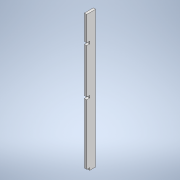
# Autodesk Inventor part: sideHolder
Saved by Autodesk Inventor 2020 (Build 240168000, 168)
## iProperties
Created: 2022-03-24
Part Number: sideHolder
Material: Pappel
Document SubType Name: Modeling
Designer: Eric
Density: 0.448 g/cm^3
Appearance: Pappel
Author: Eric
Autodesk Inventor part; units mm, degrees
ref_plane "YZ Plane" through (0, 0, 0) normal (1, 0, 0) x (0, 1, 0)
ref_plane "XZ Plane" through (0, 0, 0) normal (0, 1, 0) x (-1, 0, 0)
ref_plane "XY Plane" through (0, 0, 0) normal (0, 0, 1) x (1, 0, 0)
sketch "Skizze1" plane through (0, 0, 0) normal (1, 0, 0) x (0, 1, 0)
  line L0 (0, 0) -> (0, -15)
  line L1 (0, -15) -> (-230, -15)
  line L2 (-230, -15) -> (-230, -5)
  line L3 (-230, -5) -> (-226, -5)
  line L4 (-226, -5) -> (-226, 0)
  line L5 (-226, 0) -> (-124.5, 0)
  line L6 (-124.5, 0) -> (-124.5, -5)
  line L7 (-124.5, -5) -> (-120.5, -5)
  line L8 (-120.5, -5) -> (-120.5, 0)
  line L9 (-120.5, 0) -> (-45.5, 0)
  line L10 (-45.5, 0) -> (-45.5, -5)
  line L11 (-45.5, -5) -> (-41.5, -5)
  line L12 (-41.5, -5) -> (-41.5, 0)
  line L13 (-41.5, 0) -> (0, 0)
  dimension "d0" = 4
  dimension "d1" = 10
  dimension "d6" = 101.5
  dimension "d8" = 41.5
  dimension "d10" = 5
  dimension "d11" = 75
  constraints: 28 end point, 7 perpendicular, 7 point on line, 2 collinear, 2 horizontal, 1 vertical
  measures "d0" distance of L2.end L3.end
  measures "d1" distance between parallel lines of L1 L3
  measures "d6" distance of L4.end L5.end
  measures "d8" distance of L12.end L0.start
  measures "d10" distance of L3.end L4.end
  measures "d11" distance between parallel lines of L10 L8
extrude "Extrusion1" add sketch "Skizze1" along normal blind 4
